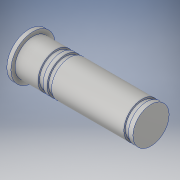
# Autodesk Inventor part: Idle pulley pin
Saved by Autodesk Inventor 2019.4 (Build 234330000, 330)
## iProperties
Created: 2020-02-23
Part Number: Idle pulley pin
Material: Aluminum 6061
Document SubType Name: Modeling
Designer: admin
Density: 2.7 g/cm^3
Appearance: Aluminum - Flat
Author: admin
Autodesk Inventor part; units mm, degrees
ref_plane "YZ Plane" through (0, 0, 0) normal (1, 0, 0) x (0, 1, 0)
ref_plane "XZ Plane" through (0, 0, 0) normal (0, 1, 0) x (-1, 0, 0)
ref_plane "XY Plane" through (0, 0, 0) normal (0, 0, 1) x (1, 0, 0)
sketch "Sketch1" plane through (0, 0, 0) normal (0, 0, 1) x (1, 0, 0)
  line L0 (0, 0) -> (0, 4.9)
  line L1 (0, 4.9) -> (0.9, 4.9)
  line L2 (0.9, 4.9) -> (0.9, 4)
  line L3 (0.9, 4) -> (6, 4)
  line L4 (6, 4) -> (6, 3.65)
  line L5 (6, 3.65) -> (7.1, 3.65)
  line L6 (7.1, 3.65) -> (7.1, 4)
  line L7 (7.1, 4) -> (8, 4)
  line L8 (8, 4) -> (8, 3.65)
  line L9 (8, 3.65) -> (9, 3.65)
  line L10 (9, 3.65) -> (9, 4)
  line L11 (9, 4) -> (25, 4)
  line L12 (25, 4) -> (25, 3.65)
  line L13 (25, 3.65) -> (26, 3.65)
  line L14 (26, 3.65) -> (26, 4)
  line L15 (26, 4) -> (27, 4)
  line L16 (27, 4) -> (27, 0)
  line L17 (27, 0) -> (0, 0)
  dimension "d0" = 0.9
  dimension "d1" = 4
  dimension "d2" = 0.9
  dimension "d3" = 1.1
  dimension "d4" = 0.35
  dimension "d5" = 1
  dimension "d6" = 1
  dimension "d7" = 1
  dimension "d8" = 16
  dimension "d9" = 5.1
  dimension "d10" = 3
  constraints: 36 end point, 12 perpendicular, 9 point on line, 1 parallel, 1 vertical
  measures "d0" distance of L0.end L1.end
  measures "d1" distance between parallel lines of L17 L3
  measures "d2" distance of L1.end L2.end
  measures "d3" distance of L4.end L5.end
  measures "d4" distance of L3.end L4.end
  measures "d5" distance of L12.end L13.end
  measures "d6" distance of L8.end L9.end
  measures "d7" distance of L14.end L15.end
  measures "d8" distance between parallel lines of L12 L10
  measures "d9" distance of L2.end L3.end
  measures "d10" distance between parallel lines of L10 L4
revolve "Revolution1" add sketch "Sketch1" angle 360 about axis through (27, 0, 0) along (-1, 0, 0)
body "Solid1"
